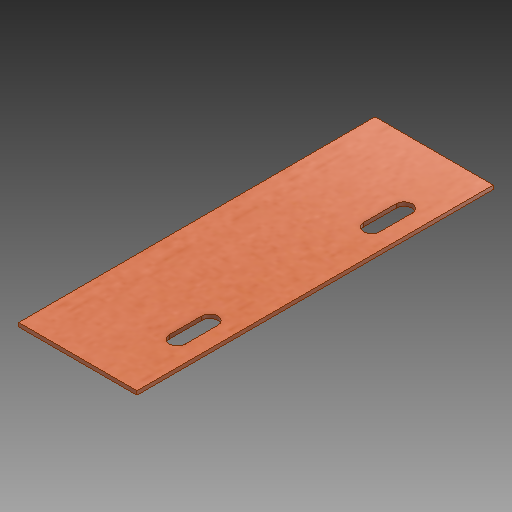
# Autodesk Inventor part: bett_V2_deckplatte_klappe
Saved by Autodesk Inventor 2018 (Build 220112000, 112)
## iProperties
Created: 2020-03-29
Part Number: bett_V2_deckplatte_klappe
Material: Holz (Walnuss)
Document SubType Name: Modeling
Designer: wepet
Density: 0.55 g/cm^3
Appearance: Walnuss - natur - poliert
Description: Sperrholzplatte 12mm - 36,5x110cm
Mass: 2.55798 g
Surface Area: 81.8876 cm^2
Volume: 4.65088 cm^3
Author: wepet
Autodesk Inventor part; units mm, degrees
ref_plane "YZ Plane" through (0, 0, 0) normal (1, 0, 0) x (0, 1, 0)
ref_plane "XZ Plane" through (0, 0, 0) normal (0, 1, 0) x (-1, 0, 0)
ref_plane "XY Plane" through (0, 0, 0) normal (0, 0, 1) x (1, 0, 0)
sketch "Skizze1" plane through (0, 0, 0) normal (0, 0, 1) x (1, 0, 0)
  line L0 (0, 0) -> (36.5, 0)
  line L1 (36.5, 0) -> (36.5, 110)
  line L2 (36.5, 110) -> (0, 110)
  line L3 (0, 110) -> (0, 91.5)
  line L4 (0, 86.5) -> (0, 91.5)
  line L5 (0, 18.5) -> (0, 23.5)
  line L6 (0, 23.5) -> (0, 18.5) construction
  line L7 (0, 18.5) -> (0, 0)
  line L8 (0, 86.5) -> (0, 23.5)
  line L9 (0, 91.5) -> (0, 86.5) construction
  line L10 (31.5, 90) -> (26.5, 90) construction
  line L11 (26.5, 90) -> (26.5, 80)
  line L12 (26.5, 80) -> (31.5, 80) construction
  line L13 (31.5, 80) -> (31.5, 90)
  line L14 (31.5, 30) -> (26.5, 30) construction
  line L15 (26.5, 30) -> (26.5, 20)
  line L16 (26.5, 20) -> (31.5, 20) construction
  line L17 (31.5, 20) -> (31.5, 30)
  line L18 (29, 80) -> (29, 30) construction
  line L19 (36.5, 55) -> (0, 55) construction
  arc A0 (31.5, 90) -> (26.5, 90) centre (29, 90) ccw
  arc A1 (26.5, 80) -> (31.5, 80) centre (29, 80) ccw
  arc A2 (31.5, 30) -> (26.5, 30) centre (29, 30) ccw
  arc A3 (26.5, 20) -> (31.5, 20) centre (29, 20) ccw
  point P0 (29, 55)
  dimension "d0" = 36.5
  dimension "d1" = 110
  dimension "d10" = 10
  dimension "d11" = 10
  dimension "d12" = 5
  dimension "d13" = 5
  dimension "d15" = 20
  constraints: 40 end point, 10 parallel, 8 point on circle, 7 midpoint, 4 centre point, 4 perpendicular, 3 horizontal, 3 point on line, 2 coincident
  measures "d0" distance of L2.end L1.end
  measures "d1" distance of L1.end L0.end
  measures "d10" distance of L12.end L10.start
  measures "d11" distance of L16.end L14.start
  measures "d12" distance of L10.start L10.end
  measures "d13" distance between parallel lines of L1 L13
  measures "d15" distance between parallel lines of L2 L10
extrude "Extrusion2" add sketch "Skizze1" along normal blind 1.2
